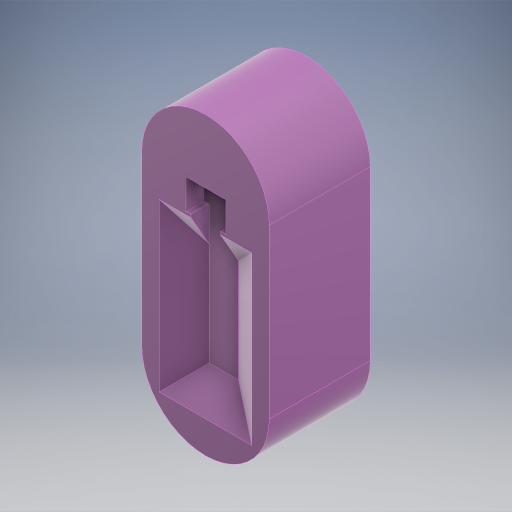
# Autodesk Inventor part: Установка датчика холла
Saved by Autodesk Inventor 2023 (Build 270158000, 158)
## iProperties
Created: 2023-03-30
Part Number: Установка датчика холла
Material: Типовые
Document SubType Name: Modeling
Designer: Admin
Density: 1 g/cm^3
Appearance: По умолчанию
Author: Admin
Autodesk Inventor part; units mm, degrees
ref_plane "YZ Plane" through (0, 0, 0) normal (1, 0, 0) x (0, 1, 0)
ref_plane "XZ Plane" through (0, 0, 0) normal (0, 1, 0) x (-1, 0, 0)
ref_plane "XY Plane" through (0, 0, 0) normal (0, 0, 1) x (1, 0, 0)
sketch "Эскиз1" plane through (0, 0, 0) normal (0, 0, 1) x (1, 0, 0)
  line L0 (-2.18, 1.65) -> (2.18, 1.65)
  line L1 (2.18, 1.65) -> (2.18, -1.65)
  line L2 (2.18, -1.65) -> (-2.18, -1.65)
  line L3 (-2.18, -1.65) -> (-2.18, 1.65)
  line L4 (-2.18, 1.65) -> (2.18, -1.65) construction
  line L5 (2.18, 1.65) -> (-2.18, -1.65) construction
  line L6 (-1.6, -1.65) -> (1.6, -1.65)
  line L7 (1.6, -1.65) -> (1.6, -16.65)
  line L8 (1.6, -16.65) -> (-1.6, -16.65)
  line L9 (-1.6, -16.65) -> (-1.6, -1.65)
  line L10 (0, 1.65) -> (0, -16.65) construction
  line L11 (-6.95, 1.65) -> (-6.95, -16.65)
  line L12 (6.95, -16.65) -> (6.95, 1.65)
  arc A0 (6.95, 1.65) -> (-6.95, 1.65) centre (0, 1.65) ccw
  arc A1 (-6.95, -16.65) -> (6.95, -16.65) centre (0, -16.65) ccw
  line L13 (-1.6, -1.65) -> (-1.6, -9.15)
  line L14 (1.6, -1.65) -> (1.6, -9.15)
  line L15 (-1.6, -5.4) -> (-5.6947, -16.65)
  line L16 (1.6, -5.4) -> (5.6947, -16.65)
  arc A2 (-5.6947, -16.65) -> (5.6947, -16.65) centre (0, -1.004) ccw
  line L17 (1.6, -5.4) -> (-1.6, -5.4)
  point P0 (0, 0)
  point P1 (0, 0)
  point P2 (0, 0)
  point P3 (0, 0)
  point P4 (0, -1.65)
  point P5 (0, 0)
  point P6 (0, -7.5)
  point P7 (1.6, -5.4)
  point P8 (-1.6, -5.4)
  point P9 (1.6, -1.65)
  dimension "d0" = 4.06
  dimension "d1" = 3
  dimension "d2" = 3.2
  dimension "d3" = 15
  dimension "d4" = 14
  dimension "d5" = 20
  dimension "d6" = 20
  constraints: 38 end point, 10 midpoint, 6 point on circle, 5 parallel, 4 coincident, 4 tangent, 3 centre point, 3 horizontal, 2 line through centre, 2 perpendicular, 1 horizontal alignment, 1 point on line, 1 vertical, 1 vertical alignment
  measures "d2" distance of L7.end L9.start
  measures "d3" distance of L7.start L7.end
  measures "d5" angle of L7 L16
  measures "d6" angle of L9 L15
extrude "Выдавливание1" add sketch "Эскиз1" along normal blind 2 and the other way blind 9 contours L0 L1 L2 L3 | L2 L7 L17 L9 | L17 L7 L8 L9 | L9 L8 L7 L16 A2 L15 | A0 L12 A1 L11
extrude "Выдавливание2" cut sketch "Эскиз1" along normal up to surface (2 mm away) draft 60 contours L17 L7 L8 L9
extrude "Выдавливание3" cut sketch "Эскиз1" along normal up to surface (2 mm away) contours L0 L1 L2 L3 | L2 L7 L17 L9
